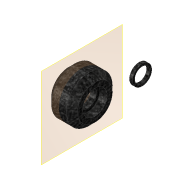
# Autodesk Inventor part: Neje_Rolls_small
Saved by Autodesk Inventor 2019.4 (Build 234330000, 330)
## iProperties
Created: 2021-04-08
Part Number: Neje_Rolls_small
Material: Generic
Document SubType Name: Modeling
Designer: diederichbenedict
Density: 1 g/cm^3
Appearance: Black Cast
Mass: 3.78382 g
Surface Area: 17.1211 cm^2
Volume: 3.78382 cm^3
Author: diederichbenedict
Autodesk Inventor part; units mm, degrees
ref_plane "YZ Plane" through (0, 0, 0) normal (1, 0, 0) x (0, 1, 0)
ref_plane "XZ Plane" through (0, 0, 0) normal (0, 1, 0) x (-1, 0, 0)
ref_plane "XY Plane" through (0, 0, 0) normal (0, 0, 1) x (1, 0, 0)
sketch "Sketch1" plane through (0, 0, 0) normal (0, 0, 1) x (1, 0, 0)
  line L0 (0, 0) -> (0, 5.85)
  line L1 (0, 0) -> (-8.8, 0)
  line L2 (-8.8, 0) -> (-8.8, 5.85)
  line L3 (-6.9, 0) -> (-6.9, 7.75)
  line L4 (-8.8, 5.85) -> (-6.9, 7.75)
  line L5 (0, 5.85) -> (-1.9, 7.75)
  line L6 (-1.9, 7.75) -> (-6.9, 7.75)
  point P0 (-5.5, 0)
  dimension "d0" = 8.8
  dimension "d1" = 7.75
  dimension "d3" = 1.9
  dimension "d8" = 5
  dimension "d9" = 45
  dimension "d10" = 135
  constraints: 14 end point, 2 horizontal, 2 point on line, 2 vertical, 1 perpendicular
  measures "d0" distance of L0.start L1.end
  measures "d1" distance of L3.start L3.end
  measures "d3" distance between parallel lines of L3 L2
  measures "d8" distance of L3.end L5.end
  measures "d9" angle of L6 L5
  measures "d10" angle of L4 L6
revolve "Revolution1" add sketch "Sketch1" angle 360 about axis through (0, 0, 0) along (-1, 0, 0)
ref_plane "Work Plane1" through (-4.4, 0, 0) normal (1, 0, 0) x (0, 0, -1)
sketch "Sketch2" plane through (0, 0, 0) normal (1, 0, 0) x (0, 0, -1)
  circle A0 centre (0, 0) radius 5.85 projected
  circle A1 centre (0, 0) radius 2.55
  point P0 (0, 0)
  dimension "d11" = 5.1
  constraints: 1 centre point, 1 coincident
  measures "d11" diameter of A1
extrude "Extrusion1" cut sketch "Sketch2" against normal through all contours A1
sketch "Sketch3" plane through (0, 0, 0) normal (0, 1, 0) x (-1, 0, 0)
  line L0 (6.9, 7.75) -> (6.9, -7.75) projected
  line L1 (8.8, 5.85) -> (8.8, -5.85) projected
  line L2 (8.8, 0) -> (6.3, 0)
  line L3 (6.3, 0) -> (6.3, -4.1)
  line L4 (6.3, -4.1) -> (8.8, -4.1)
  line L5 (8.8, -4.1) -> (8.8, 0)
  line L6 (0, 0) -> (2.5, 0)
  line L7 (2.5, 0) -> (2.5, -4.1)
  line L8 (2.5, -4.1) -> (0, -4.1)
  line L9 (0, -4.1) -> (0, 0)
  line L10 (6.3, 0) -> (2.5, 0)
  line L11 (2.5, 0) -> (2.5, -3.0215)
  line L12 (2.5, -3.0215) -> (6.3, -3.0215)
  line L13 (6.3, -3.0215) -> (6.3, 0)
  dimension "d14" = 2.5
  dimension "d15" = 4.1
  dimension "d16" = 2.5
  constraints: 24 end point, 6 parallel, 3 horizontal, 3 perpendicular, 2 point on line, 1 midpoint
  measures "d14" distance of L4.end L3.end
  measures "d15" distance of L3.end L2.end
  measures "d16" distance of L7.end L8.end
revolve "Revolution2" cut sketch "Sketch3" angle 360 about axis through (-6.3, 0, 0) along (1, 0, 0)
sketch "Sketch4" plane through (0, 0, 0) normal (1, 0, 0) x (0, 0, -1)
  circle A0 centre (15.8512, 0) radius 2.5
  circle A1 centre (15.8512, 0) radius 3.25
  point P0 (0, 0)
  dimension "d18" = 5
  dimension "d19" = 6.5
  constraints: 2 centre point, 1 coincident
  measures "d18" diameter of A0
  measures "d19" diameter of A1
extrude "Extrusion2" add sketch "Sketch4" against normal blind 1
body "Solid1"
